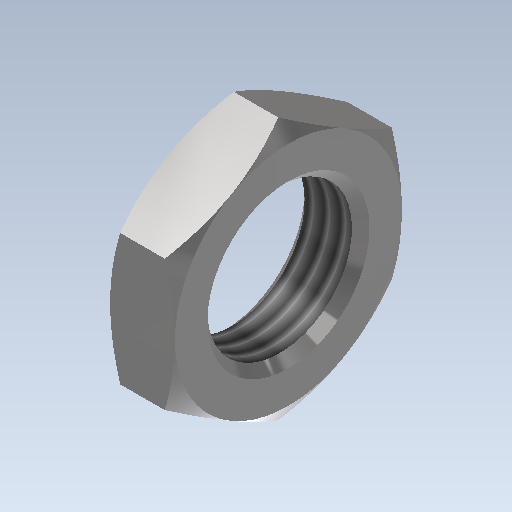
# Autodesk Inventor part: CJ2K10Z_NUT
Saved by Autodesk Inventor 2021.3 (Build 253353010, 353A)
## iProperties
Created: 2019-10-24
Part Number: CJ2K10Z_NUT
Material: ステンレス鋼
Catalog Web Link: www.cadenas.de
Description: CJ2K-Z_NUT-Air Cylinder/Non-rotating Rod Type: Double Acting, Single Rod
Vendor: SMC
Document SubType Name: Modeling
Designer: psadmin
Manufacturer: SMC
Mass: 3.3173 g
Surface Area: 4.87707 cm^2
Volume: 0.414663 cm^3
Density: 8 g/cm^3
Appearance: 半つや出し
Category: PARTsolutions
Company: SMC
PSOL_IDENT_0: {$CADENAS_DATA\23d-libs\smc_jp\actuator\standard_air_cylinder\cj2\cj2k_z\parts\cj2k_z_nut.prj},166 {
PSOL_IDENT_1: VTYP=3D},{NB=CJ2K10Z_NUT},{LINA=CJ2K10Z_NUT},{NN=CJ2K-Z_NUT},{DATE=07.02.2019 07:32:00},{GEOMDATE=12
PSOL_IDENT_2: .08.2013 00:00:00},{VERSION=},{LINEID=10},{WBVAR=},{WBNUMERIC=}  {NB=CJ2K10Z_NUT},{LINA=CJ2K10Z_NUT}
PSOL_IDENT_3: ,{KT=DUMMY},{BORE=10.000},{NN=M10x1},{NNA=10.000},{NNP=1.000},{H=14.000},{D=4.000}
NN: M10x1
NT: Air Cylinder/Non-rotating Rod Type: Double Acting, Single Rod
NB: CJ2K10Z_NUT
NBSYN: CJ2K$BORE.Z_NUT
LINA: CJ2K10Z_NUT
BORE: 10
NNA: 10
NNP: 1
H: 14
D: 4
SUPPLIER: SMC
ARTICLENO: CJ2K10Z_NUT
BOMINFO: CJ2K10Z_NUT
CREATOR: CADENAS GmbH
Title: CJ2K10Z_NUT
Author: Cadenas PARTsolutions
Comments: Air Cylinder/Non-rotating Rod Type: Double Acting, Single Rod
Autodesk Inventor part; units mm, degrees
sketch "Sketch_1" plane through (0, 0, 0) normal (0, 0, 1) x (1, 0, 0)
  line L0 (50, 0) -> (-50, 0)
  line L1 (0, 7) -> (0, 5)
  line L2 (0, 5) -> (0.5415, 4.4585)
  line L3 (0.5415, 4.4585) -> (3.4585, 4.4585)
  line L4 (3.4585, 4.4585) -> (4, 5)
  line L5 (4, 5) -> (4, 7)
  line L6 (4, 7) -> (2.3834, 9.8)
  line L7 (2.3834, 9.8) -> (1.6166, 9.8)
  line L8 (1.6166, 9.8) -> (0, 7)
  constraints: 18 end point
revolve "Revolution1" add sketch "Sketch_1" angle 360 about axis through (50, 0, 0) along (1, 0, 0)
thread "Thread1" size "M10x1" class "6H" standard "ISO Metric profile" full length
sketch "Sketch_2" plane through (0, 0, 0) normal (1, 0, 0) x (0, 1, 0)
  circle A0 centre (0, 0) radius 14
  line L0 (-4.0415, 7) -> (-8.0829, 0)
  line L1 (-8.0829, 0) -> (-4.0415, -7)
  line L2 (-4.0415, -7) -> (4.0415, -7)
  line L3 (4.0415, -7) -> (8.0829, 0)
  line L4 (8.0829, 0) -> (4.0415, 7)
  line L5 (4.0415, 7) -> (-4.0415, 7)
  constraints: 12 end point, 1 centre point
extrude "Extrusion1" cut sketch "Sketch_2" along normal blind 4
ref_plane "NUT_XY" through (0, 0, 0) normal (1, 0, 0) x (0, 0, -1)
ref_plane "NUT_YZ" through (0, 0, 0) normal (0, 0, -1) x (0, 1, 0)
ref_plane "NUT_ZX" through (0, 0, 0) normal (0, 1, 0) x (1, 0, 0)
body "Solid1"
